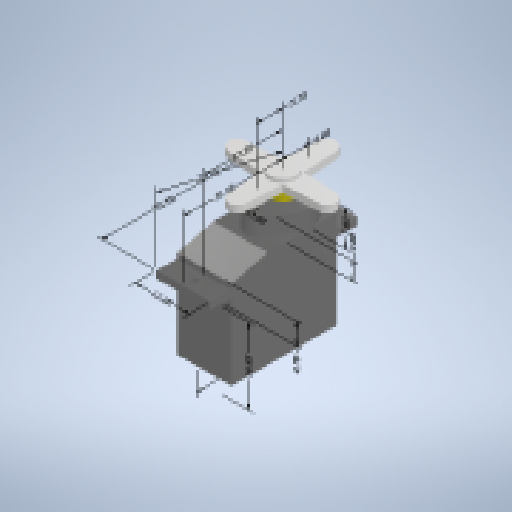
# Autodesk Inventor part: FT90MR
Saved by Autodesk Inventor 2024.1 (Build 281209000, 209)
## iProperties
Created: 2024-11-26
Part Number: FT90MR
Material: ABS プラスチック
Document SubType Name: Modeling
Designer: hibik
Density: 1.06 g/cm^3
Appearance: ゴム - 黒 - バージョン 1.1
Author: hibik
Autodesk Inventor part; units mm, degrees
ref_plane "YZ Plane" through (0, 0, 0) normal (1, 0, 0) x (0, 1, 0)
ref_plane "XZ Plane" through (0, 0, 0) normal (0, 1, 0) x (-1, 0, 0)
sketch "スケッチ1" plane through (0, 0, 0) normal (0, 1, 0) x (-1, 0, 0)
  line L0 (0, 0) -> (12, 0)
  line L1 (12, 0) -> (12, -23.3)
  line L2 (12, -23.3) -> (0, -23.3)
  line L3 (0, -23.3) -> (0, 0)
  dimension "d0" = 23.3
  dimension "d1" = 12
  constraints: 8 end point, 2 parallel, 1 horizontal, 1 perpendicular
  measures "d0" distance of L0.end L1.end
  measures "d1" distance of L1.end L2.end
extrude "押し出し1" add sketch "スケッチ1" along normal blind 18.45
sketch "スケッチ2" plane through (0, 18.45, 0) normal (0, 1, 0) x (1, 0, 0)
  circle A0 centre (-6, 17.3) radius 6
  line L0 (-12, 23.3) -> (-12, 0)
  line L1 (0, 0) -> (0, 23.3)
  line L2 (0, 23.3) -> (-12, 23.3)
  circle A1 centre (-6, 11.6) radius 2.5
  line L3 (-7.973197, 10.064912) -> (-10.735672, 13.615789)
  line L4 (-4.026803, 10.064912) -> (-1.264328, 13.615789)
  point P0 (-8.488419, 11.840351)
  point P1 (-3.511581, 11.840351)
  dimension "d20" = 5.7
  dimension "d21" = 5
  constraints: 7 tangent, 4 end point, 4 point on circle, 2 centre point, 1 vertical alignment
  measures "d20" distance of A0.centre A1.centre
  measures "d21" diameter of A1
extrude "押し出し2" add sketch "スケッチ2" along normal blind 6.9 contours A0 A1 | L4 A1 A0 | A1 A0 | A0 A1 | A1 L3 A0
sketch "スケッチ3" plane through (-6, 25.35, -17.3) normal (0, 1, 0) x (-1, 0, 0)
  arc A0 (-4.735672, 3.684211) -> (4.735672, 3.684211) centre (0, 0) ccw
  circle A1 centre (0, 0) radius 2.5
  point P0 (-6, 17.3)
  point P1 (-2.386497, 4.955263)
  point P2 (2.386497, 4.955263)
  dimension "d6" = 5
  constraints: 1 centre point, 1 coincident
  measures "d6" diameter of A1
extrude "押し出し3" add sketch "スケッチ3" along normal blind 3.1
sketch "スケッチ4" plane through (0, 18.45, 0) normal (0, 1, 0) x (1, 0, 0)
  line L0 (0, 0) -> (0, 23.3) projected
  line L1 (0, 17.3) -> (0, 23.3) projected
  line L2 (0, 0) -> (0, 17.3) projected
  line L3 (0, 23.3) -> (-12, 23.3) projected
  line L4 (0, 0) -> (0, 23.3) projected
  line L5 (-12, 0) -> (0, 0) projected
  line L6 (-12, 23.3) -> (-12, 0) projected
  line L7 (-12, -4.6) -> (0, -4.6)
  line L8 (0, -4.6) -> (0, 27.9)
  line L9 (0, 27.9) -> (-12, 27.9)
  line L10 (-12, 27.9) -> (-12, -4.6)
  line L11 (-12, -2.6) -> (0, -2.6) construction
  line L12 (0, -2.6) -> (0, 25.9) construction
  line L13 (0, 25.9) -> (-12, 25.9) construction
  line L14 (-12, 25.9) -> (-12, -2.6) construction
  line L15 (0, 17.3) -> (0, 23.3) projected
  circle A0 centre (-6, -2.6) radius 0.85
  circle A1 centre (-6, 25.9) radius 0.85
  point P0 (-12, 11.65)
  point P1 (-12, 23.3)
  dimension "d9" = 32.5
  dimension "d10" = 28.5
  dimension "d11" = 1.7
  dimension "d12" = 1.7
  constraints: 16 end point, 5 midpoint, 4 parallel, 2 centre point, 2 collinear, 2 horizontal, 2 perpendicular
  measures "d9" distance of L9.end L7.start
  measures "d10" distance of L13.end L11.start
  measures "d11" diameter of A0
  measures "d12" diameter of A1
extrude "押し出し4" add sketch "スケッチ4" against normal blind 1.6 contours L8 L7 L10 L5 | L3 L10 L9 L8
sketch "スケッチ5" plane through (0, 18.45, 0) normal (0, 1, 0) x (1, 0, 0)
  line L0 (0, 23.3) -> (-12, 23.3) projected
  line L1 (0, 0) -> (0, 23.3) projected
  line L2 (-12, 0) -> (0, 0) projected
  line L3 (-12, 23.3) -> (-12, 0) projected
extrude "押し出し5" add sketch "スケッチ5" along normal blind 3.1
chamfer "面取り1" distance 8 distance2 2 1 edges at (-6, 21.55, 0) measured on face at (-6, 21.55, -3.0333)
ref_plane "作業平面1" through (0, 29.35, 0) normal (0, 1, 0) x (1, 0, 0)
sketch "スケッチ6" plane through (0, 29.35, 0) normal (0, 1, 0) x (1, 0, 0)
  circle A0 centre (-6, 17.3) radius 2.5
  circle A1 centre (-6, 17.3) radius 11.9
  circle A2 centre (-6, 27.2) radius 2
  circle A3 centre (-15.9, 17.3) radius 2
  circle A4 centre (-6, 7.4) radius 2
  circle A5 centre (3.9, 17.3) radius 2
  line L0 (4.00101, 19.297448) -> (-5.873737, 19.79681)
  line L1 (-5.873737, 14.80319) -> (4.00101, 15.302552)
  line L2 (-7.997448, 27.30101) -> (-8.49681, 17.426263)
  line L3 (-3.50319, 17.426263) -> (-4.002552, 27.30101)
  line L4 (-16.00101, 15.302552) -> (-6.126263, 14.80319)
  line L5 (-6.126263, 19.79681) -> (-16.00101, 19.297448)
  line L6 (-4.002552, 7.29899) -> (-3.50319, 17.173737)
  line L7 (-8.49681, 17.173737) -> (-7.997448, 7.29899)
  point P0 (0, 0)
  point P1 (-8.382702, 14.917298)
  point P2 (-7.997448, 7.29899)
  point P3 (-4.002552, 7.29899)
  point P4 (-3.617298, 14.917298)
  point P5 (-3.617298, 19.682702)
  point P6 (-4.002552, 27.30101)
  point P7 (-7.997448, 27.30101)
  point P8 (-8.382702, 19.682702)
  point P9 (-16.00101, 19.297448)
  dimension "d34" = 23.8
  dimension "d35" = 4
  dimension "d38" = 360
  dimension "d42" = 360
  constraints: 16 end point, 5 centre point, 5 tangent, 4 point on circle, 1 coincident, 1 vertical alignment, 34 other
  measures "d34" diameter of A1
  measures "d35" diameter of A2
sketch "スケッチ6 outline for 押し出し6" plane through (0, 29.35, 0) normal (0, 1, 0) x (1, 0, 0)
  line L0 (-8.382702, 14.917298) -> (-7.997448, 7.29899)
  arc A0 (-7.997448, 7.29899) -> (-4.002552, 7.29899) centre (-6, 7.4) ccw
  line L1 (-4.002552, 7.29899) -> (-3.617298, 14.917298)
  line L2 (-3.617298, 14.917298) -> (4.00101, 15.302552)
  arc A1 (4.00101, 15.302552) -> (4.00101, 19.297448) centre (3.9, 17.3) ccw
  line L3 (4.00101, 19.297448) -> (-3.617298, 19.682702)
  line L4 (-3.617298, 19.682702) -> (-4.002552, 27.30101)
  arc A2 (-4.002552, 27.30101) -> (-7.997448, 27.30101) centre (-6, 27.2) ccw
  line L5 (-7.997448, 27.30101) -> (-8.382702, 19.682702)
  line L6 (-8.382702, 19.682702) -> (-16.00101, 19.297448)
  arc A3 (-16.00101, 19.297448) -> (-16.00101, 15.302552) centre (-15.9, 17.3) ccw
  line L7 (-16.00101, 15.302552) -> (-8.382702, 14.917298)
extrude "押し出し6" add sketch "スケッチ6 outline for 押し出し6" against normal blind 1.6
sketch "スケッチ7" plane through (0, 29.35, 0) normal (0, 1, 0) x (1, 0, 0)
  circle A0 centre (-6, 17.3) radius 2.5 projected
  circle A1 centre (-6, 17.3) radius 2.95
  point P0 (0, 0)
  dimension "d46" = 5.9
  constraints: 1 centre point, 1 coincident
  measures "d46" diameter of A1
extrude "押し出し7" add sketch "スケッチ7" along normal blind 0.8 contours A0 | A1
